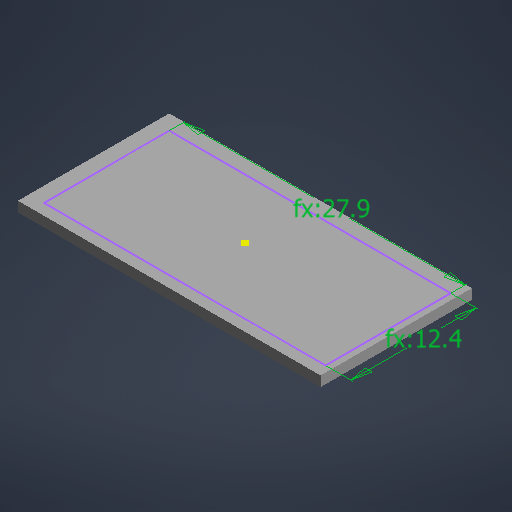
# Autodesk Inventor part: tray_multipart
Saved by Autodesk Inventor 2026 (Build 300175050, 175E)
## iProperties
Part Number: tray_multipart
Material: Generic
Document SubType Name: Modeling
Designer: romanov
Appearance: Default
Author: romanov
Autodesk Inventor part; units mm, degrees
ref_plane "YZ Plane" through (0, 0, 0) normal (1, 0, 0) x (0, 1, 0)
ref_plane "XZ Plane" through (0, 0, 0) normal (0, 1, 0) x (-1, 0, 0)
ref_plane "XY Plane" through (0, 0, 0) normal (0, 0, 1) x (1, 0, 0)
sketch "Sketch1" plane through (0, 0, 0) normal (0, 1, 0) x (-1, 0, 0)
  line L0 (150, 75) -> (-150, 75)
  line L1 (-150, 75) -> (-150, -75)
  line L2 (-150, -75) -> (150, -75)
  line L3 (150, -75) -> (150, 75)
  line L4 (150, 75) -> (-150, -75) construction
  line L5 (-150, 75) -> (150, -75) construction
  point P0 (0, 0)
  dimension "d0" = 300
  dimension "d1" = 150
  constraints: 12 end point, 2 midpoint, 2 parallel, 1 horizontal, 1 perpendicular
  measures "d0" distance between parallel lines of L1 L3
  measures "d1" distance between parallel lines of L0 L2
extrude "Extrusion1" add sketch "Sketch1" along normal blind 10
sketch "Sketch2" plane through (0, 10, 0) normal (0, 1, 0) x (1, 0, 0)
  point P0 (0, 0)
sketch "Sketch3" plane through (0, 10, 0) normal (0, 1, 0) x (1, 0, 0)
  line L0 (-135.1051, -63.9197) -> (143.8949, -63.9197)
  line L1 (143.8949, -63.9197) -> (143.8949, 60.0803)
  line L2 (143.8949, 60.0803) -> (-135.1051, 60.0803)
  line L3 (-135.1051, 60.0803) -> (-135.1051, -63.9197)
  point P0 (0, 0)
  dimension "d4" = 279
  dimension "d5" = 124
  constraints: 8 end point, 2 parallel, 1 horizontal, 1 perpendicular
  measures "d4" distance of L1.end L2.end
  measures "d5" distance of L0.end L1.end
equation "\"d4\" = pebble_width"
equation "\"d5\" = pebble_height"
equation "\"pebble_height\" = 124"
equation "\"pebble_width\" = 279"
equation "\"pebble_depth\" = 16"
body "Solid1"
